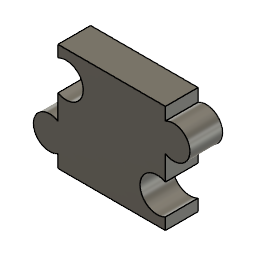
Platform (Autodesk Fusion 360 archive; units mm, degrees)
design "Platform"
part number: Center
Autodesk Fusion 360 part; units mm, degrees
sketch "Platform" plane through (0, 0, 0) normal (0, 1, 0) x (1, 0, 0)
  line L0 (0, -53) -> (0, -45)
  line L1 (26.25, -45) -> (0, -45)
  line L2 (26.25, -53) -> (0, -53)
  line L3 (26.25, -45) -> (26.25, -53)
  dimension "d2" = 26.25
  dimension "d3" = 45
  dimension "d68" = 8
  constraint vertical L3
  constraint horizontal L2
  constraint vertical L0
  constraint coincident origin L0
  constraint horizontal L1
  constraint coincident L0.end L1.end
  constraint coincident L1.start L3.start
  measures "d2" distance of L0 L3
  measures "d3" distance of origin L1
  measures "d68" distance of L1 L2
extrude "Extrude1" add sketch "Platform" along normal mid plane 26.25
sketch "Puzzle" plane through (0, 0, 45) normal (0, 0, -1) x (-1, 0, 0)
  circle A0 centre (-2, 6.5625) radius 4.2
  line L0 (0, -13.125) -> (-26.25, 0) construction
  line L1 (-13.125, -13.125) -> (-13.125, 0) construction
  circle A1 centre (2, 6.5625) radius 4 construction
  line L2 (-24.25, -10.7625) -> (-24.25, -2.3625) construction
  circle A2 centre (-24.25, -6.5625) radius 4.2
  circle A3 centre (-24.25, 6.5625) radius 4.2 construction
  circle A4 centre (-24.25, -6.5625) radius 4 construction
  line L3 (0, 0) -> (-26.25, 0) construction
  line L4 (0, 0) -> (-26.25, -13.125) construction
  circle A5 centre (-28.25, 6.5625) radius 4
  circle A6 centre (2, -6.5625) radius 4
  line L5 (2, -10.5625) -> (2, -2.5625) construction
  line L6 (-26.25, 13.125) -> (-26.25, -13.125)
  line L7 (0, -13.125) -> (0, 13.125)
  line L8 (0, 13.125) -> (-26.25, 13.125)
  line L9 (-26.25, 13.125) -> (-26.25, -13.125)
  line L10 (-26.25, -13.125) -> (0, -13.125)
  point P0 (-13.125, -6.5625)
  dimension "d11" = 8
  dimension "d13" = 2
  dimension "d14" = 0.2
  dimension "d83" = 2
  constraint coincident L5.start A6
  constraint coincident L5.end A6
  constraint vertical L5
  constraint coincident A6.centre L5
  constraint coincident L3.start L4.start
  constraint coincident L0.end L6
  constraint horizontal L3
  constraint coincident L4.end L6.end
  constraint midpoint P0 L0
  constraint horizontal P0 A6.centre
  constraint midpoint L1.end L3
  constraint coincident L2.start A2
  constraint coincident L2.end A2
  constraint vertical L2
  constraint coincident A2.centre L2
  constraint horizontal A2.centre P0
  constraint symmetric A2 A3 L3
  constraint symmetric A0 L1 A3
  constraint symmetric A1 L3 A6
  constraint symmetric L1 A1 A5
  constraint equal A4 A6
  constraint coincident A2.centre A4.centre
  constraint coincident L4.start L3
  constraint coincident L6.start L8.end
  constraint coincident L0.start L7.start
  constraint coincident L1.start L10
  constraint vertical L1
  measures "d11" diameter of A6
  measures "d13" distance of L2 L6
  measures "d14" distance of A2 A4
  measures "d83" distance of L5 L7
sketch "Pillar" plane through (0, 0, 45) normal (0, 0, -1) x (-1, 0, 0)
  line L0 (0, -13.125) -> (0, 13.125)
  line L1 (0, 13.125) -> (-26.25, 13.125)
  line L2 (-26.25, 13.125) -> (-26.25, -13.125)
  line L3 (-26.25, -13.125) -> (0, -13.125)
  line L4 (-11.125, 1) -> (-15.125, 1)
  line L5 (-15.125, 1) -> (-15.125, -1)
  line L6 (-15.125, -1) -> (-11.125, -1)
  line L7 (-11.125, -1) -> (-11.125, 1)
  line L8 (-11.125, 1) -> (-15.125, -1) construction
  line L9 (-15.125, 1) -> (-11.125, -1) construction
  line L10 (-11.325, 0.8) -> (-14.925, 0.8)
  line L11 (-14.925, 0.8) -> (-14.925, -0.8)
  line L12 (-14.925, -0.8) -> (-11.325, -0.8)
  line L13 (-11.325, -0.8) -> (-11.325, 0.8)
  line L14 (-11.325, 0.8) -> (-14.925, -0.8) construction
  line L15 (-14.925, 0.8) -> (-11.325, -0.8) construction
  line L16 (-17.325, 0.8) -> (-20.925, 0.8)
  line L17 (-17.325, 0.8) -> (-20.925, -0.8) construction
  line L18 (-21.125, 1) -> (-17.125, -1) construction
  line L19 (-17.125, -1) -> (-17.125, 1)
  line L20 (-20.925, 0.8) -> (-17.325, -0.8) construction
  line L21 (-17.325, -0.8) -> (-17.325, 0.8)
  line L22 (-21.125, 1) -> (-21.125, -1)
  line L23 (-17.125, 1) -> (-21.125, 1)
  line L24 (-17.125, 1) -> (-21.125, -1) construction
  line L25 (-21.125, -1) -> (-17.125, -1)
  line L26 (-20.925, 0.8) -> (-20.925, -0.8)
  line L27 (-20.925, -0.8) -> (-17.325, -0.8)
  line L28 (-5.325, 0.8) -> (-8.925, 0.8)
  line L29 (-5.325, 0.8) -> (-8.925, -0.8) construction
  line L30 (-9.125, 1) -> (-5.125, -1) construction
  line L31 (-5.125, -1) -> (-5.125, 1)
  line L32 (-8.925, 0.8) -> (-5.325, -0.8) construction
  line L33 (-5.325, -0.8) -> (-5.325, 0.8)
  line L34 (-9.125, 1) -> (-9.125, -1)
  line L35 (-5.125, 1) -> (-9.125, 1)
  line L36 (-5.125, 1) -> (-9.125, -1) construction
  line L37 (-9.125, -1) -> (-5.125, -1)
  line L38 (-8.925, 0.8) -> (-8.925, -0.8)
  line L39 (-8.925, -0.8) -> (-5.325, -0.8)
  circle A0 centre (-13.125, 0) radius 13.125 construction
  point P0 (-13.125, 0)
  point P1 (-13.125, 0)
  point P2 (-19.125, 0)
  point P3 (-19.125, 0)
  point P4 (-7.125, 0)
  point P5 (-7.125, 0)
  dimension "d69" = 4
  dimension "d70" = 2
  dimension "d71" = 0.2
  dimension "d72" = 0.2
  dimension "d73" = 4
  dimension "d74" = 2
  dimension "d75" = 0.2
  dimension "d76" = 0.2
  dimension "d77" = 4
  dimension "d78" = 2
  dimension "d79" = 0.2
  dimension "d80" = 0.2
  dimension "d81" = 6
  dimension "d82" = 6
  constraint horizontal L4
  constraint perpendicular L4 L5
  constraint parallel L4 L6
  constraint parallel L5 L7
  constraint coincident L8 P1
  constraint coincident L9 P1
  constraint horizontal L10
  constraint perpendicular L10 L11
  constraint parallel L10 L12
  constraint parallel L11 L13
  constraint coincident L14 P1
  constraint coincident L15 P1
  constraint coincident P1 P0
  constraint horizontal L23
  constraint perpendicular L22 L23
  constraint parallel L23 L25
  constraint parallel L19 L22
  constraint coincident P3 L24
  constraint coincident P3 L18
  constraint horizontal L16
  constraint perpendicular L16 L26
  constraint parallel L16 L27
  constraint parallel L21 L26
  constraint coincident P3 L17
  constraint coincident P3 L20
  constraint coincident P3 P2
  constraint horizontal L35
  constraint perpendicular L34 L35
  constraint parallel L35 L37
  constraint parallel L31 L34
  constraint coincident P5 L36
  constraint coincident P5 L30
  constraint horizontal L28
  constraint perpendicular L28 L38
  constraint parallel L28 L39
  constraint parallel L33 L38
  constraint coincident P5 L29
  constraint coincident P5 L32
  constraint coincident P5 P4
  constraint horizontal origin P1
  constraint tangent L0 A0
  constraint tangent L2 A0
  constraint horizontal origin P5
  constraint horizontal origin P3
  measures "d69" distance of L5 L7
  measures "d70" distance of L4 L6
  measures "d71" distance of L4 L10
  measures "d72" distance of L7 L13
  measures "d73" distance of L19 L22
  measures "d74" distance of L23 L25
  measures "d75" distance of L16 L23
  measures "d76" distance of L19 L21
  measures "d77" distance of L31 L34
  measures "d78" distance of L35 L37
  measures "d79" distance of L28 L35
  measures "d80" distance of L31 L33
  measures "d81" distance of P1 P5
  measures "d82" distance of P1 P3
extrude "Extrude13" cut sketch "Pillar" against normal blind 2 contours L4 L5 L6 L7 | L10 L11 L12 L13 | L16 L21 L26 L27 | L19 L22 L23 L25 | L28 L33 L38 L39 | L31 L34 L35 L37
extrude "PuzzleHoleLeft" cut sketch "Puzzle" against normal up to surface (8 mm away) contours A0 L7 picked at (-2.0667, 6.5625)
extrude "PuzzleHoleRight" cut sketch "Puzzle" against normal up to surface (8 mm away) contours A2 L6 L9 picked at (-24.0556, -6.0704)
extrude "PuzzleStumpLeft" add sketch "Puzzle" against normal up to surface (8 mm away) contours A6 L7 picked at (1.8236, -5.5691)
extrude "PuzzleStumpRight" add sketch "Puzzle" against normal blind 8 contours A5 L6 L9 picked at (-28.2351, 6.3638)
equation "d2 = LetterWidth"
equation "d3 = PlatformOffset"
equation "PlatformOffset = 45 mm"
equation "PlatformHeight = 8 mm"
equation "LetterWidth = 26.25 mm"
equation "d9 = LetterWidth"
equation "d11 = PuzzleRadius"
equation "d13 = PuzzleOffset"
equation "d14 = Gap"
equation "PuzzleOffset = 2 mm"
equation "PuzzleRadius = 8 mm"
equation "Gap = 0.2 mm"
equation "d45 = -PlatformHeight"
equation "PillarWidth = 4 mm"
equation "PillarHeight = 2 mm"
equation "PillarDepth = 2 mm"
equation "PillarSpread = 6 mm"
equation "d68 = PlatformHeight"
equation "d69 = PillarWidth"
equation "d70 = PillarHeight"
equation "d71 = Gap"
equation "d72 = Gap"
equation "d73 = PillarWidth"
equation "d74 = PillarHeight"
equation "d75 = Gap"
equation "d76 = Gap"
equation "d77 = PillarWidth"
equation "d78 = PillarHeight"
equation "d79 = Gap"
equation "d80 = Gap"
equation "d81 = PillarSpread"
equation "d82 = PillarSpread"
equation "d83 = PuzzleOffset"
equation "d84 = -PillarDepth"
named bodies: "Platform"
